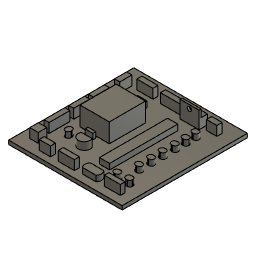
BIOGASMONITORING cad v0 (Autodesk Fusion 360 design; units mm, degrees)
Autodesk Fusion 360 part; units mm, degrees
sketch "Sketch1" plane through (0, 0, 0) normal (0, 1, 0) x (1, 0, 0)
  line L0 (25, 75) -> (85.032, 75)
  line L1 (85.032, 75) -> (85.032, 8.776)
  line L2 (85.032, 8.776) -> (25, 8.776)
  line L3 (25, 8.776) -> (25, 75)
  dimension "d1" = 60.032
  dimension "d2" = 66.224
  constraint horizontal L0
  constraint vertical L1
  constraint horizontal L2
  constraint vertical L3
  measures "d1" distance of L0.start L0.end
  measures "d2" distance of L0.start L2.end
extrude "Extrude1" add sketch "Sketch1" along normal blind 2
sketch "Sketch2" plane through (0, 2, 0) normal (0, 1, 0) x (-1, 0, 0)
  line L0 (-25, -8.776) -> (-85.032, -8.776)
  line L1 (-85.032, -8.776) -> (-85.032, -75)
  line L2 (-85.032, -75) -> (-25, -75)
  line L3 (-25, -75) -> (-25, -8.776)
  line L4 (-35.9338, -68.308) -> (-44.4138, -68.308)
  line L5 (-44.4138, -68.308) -> (-44.4138, -65.648)
  line L6 (-44.4138, -65.648) -> (-35.9338, -65.648)
  line L7 (-35.9338, -65.648) -> (-35.9338, -68.308)
  line L8 (-48.4167, -68.308) -> (-59.4367, -68.308)
  line L9 (-59.4367, -68.308) -> (-59.4367, -65.648)
  line L10 (-59.4367, -65.648) -> (-48.4167, -65.648)
  line L11 (-48.4167, -65.648) -> (-48.4167, -68.308)
  line L12 (-60.3881, -68.308) -> (-70.3881, -68.308)
  line L13 (-70.3881, -68.308) -> (-70.3881, -63.808)
  line L14 (-70.3881, -63.808) -> (-60.3881, -63.808)
  line L15 (-60.3881, -63.808) -> (-60.3881, -68.308)
  line L16 (-72.8571, -68.308) -> (-78.3401, -68.308)
  line L17 (-78.3401, -68.308) -> (-78.3401, -65.508)
  line L18 (-78.3401, -65.508) -> (-72.8571, -65.508)
  line L19 (-72.8571, -65.508) -> (-72.8571, -68.308)
  constraint horizontal L4
  constraint vertical L5
  constraint horizontal L6
  constraint vertical L7
  constraint horizontal L8
  constraint vertical L9
  constraint horizontal L10
  constraint vertical L11
  constraint horizontal L12
  constraint vertical L13
  constraint horizontal L14
  constraint vertical L15
  constraint horizontal L16
  constraint vertical L17
  constraint horizontal L18
  constraint vertical L19
extrude "Extrude2" add sketch "Sketch2" along normal blind 5 contours L4 L5 L6 L7 | L8 L9 L10 L11 | L16 L17 L18 L19
sketch "Sketch3" plane through (0, 2, 0) normal (0, 1, 0) x (-1, 0, 0)
  line L0 (-72.8571, -65.508) -> (-72.8571, -68.308)
  line L1 (-72.8571, -68.308) -> (-78.3401, -68.308)
  line L2 (-78.3401, -68.308) -> (-78.3401, -65.508)
  line L3 (-78.3401, -65.508) -> (-72.8571, -65.508)
  line L4 (-35.9338, -65.648) -> (-35.9338, -68.308)
  line L5 (-35.9338, -68.308) -> (-44.4138, -68.308)
  line L6 (-44.4138, -68.308) -> (-44.4138, -65.648)
  line L7 (-44.4138, -65.648) -> (-35.9338, -65.648)
  line L8 (-48.4167, -65.648) -> (-48.4167, -68.308)
  line L9 (-48.4167, -68.308) -> (-59.4367, -68.308)
  line L10 (-59.4367, -68.308) -> (-59.4367, -65.648)
  line L11 (-59.4367, -65.648) -> (-48.4167, -65.648)
  line L12 (-25, -8.776) -> (-85.032, -8.776)
  line L13 (-85.032, -8.776) -> (-85.032, -75)
  line L14 (-85.032, -75) -> (-25, -75)
  line L15 (-25, -75) -> (-25, -8.776)
  line L16 (-60.5977, -68.308) -> (-70.5977, -68.308)
  line L17 (-70.5977, -68.308) -> (-70.5977, -63.808)
  line L18 (-70.5977, -63.808) -> (-60.5977, -63.808)
  line L19 (-60.5977, -63.808) -> (-60.5977, -68.308)
  line L20 (-60.5977, -65.0802) -> (-70.5977, -65.0802)
  constraint horizontal L16
  constraint vertical L17
  constraint horizontal L18
  constraint vertical L19
  constraint coincident L19 L20.start
  constraint coincident L17 L20.end
  constraint perpendicular L17 L20
extrude "Extrude3" add sketch "Sketch3" along normal blind 5 contours L16 L17 L19 L20 | L17 L18 L19 L20
sketch "Sketch4" plane through (0, 7, 0) normal (0, 1, 0) x (-1, 0, 0)
  line L0 (-60.5977, -63.808) -> (-70.5977, -63.808)
  line L1 (-70.5977, -63.808) -> (-70.5977, -68.308)
  line L2 (-70.5977, -68.308) -> (-60.5977, -68.308)
  line L3 (-60.5977, -68.308) -> (-60.5977, -63.808)
  line L4 (-60.5977, -64.9469) -> (-70.5977, -64.9469)
  constraint coincident L3 L4.start
  constraint coincident L1 L4.end
  constraint perpendicular L1 L4
extrude "Extrude4" add sketch "Sketch4" along normal blind 4 contours L0 L1 L3 L4
sketch "Sketch5" plane through (0, 0, -64.9469) normal (0, 0, -1) x (-1, 0, 0)
  line L0 (-70.5977, 7) -> (-60.5977, 7)
  line L1 (-60.5977, 7) -> (-60.5977, 11)
  line L2 (-60.5977, 11) -> (-70.5977, 11)
  line L3 (-70.5977, 11) -> (-70.5977, 7)
  circle A0 centre (-65.5, 9) radius 1.118
extrude "Extrude5" cut sketch "Sketch5" against normal blind 1.5 contours A0
sketch "Sketch6" plane through (0, 2, 0) normal (0, 1, 0) x (-1, 0, 0)
  line L0 (-60.5977, -63.808) -> (-60.5977, -68.308)
  line L1 (-60.5977, -68.308) -> (-70.5977, -68.308)
  line L2 (-70.5977, -68.308) -> (-70.5977, -63.808)
  line L3 (-70.5977, -63.808) -> (-60.5977, -63.808)
  line L4 (-72.8571, -65.508) -> (-72.8571, -68.308)
  line L5 (-72.8571, -68.308) -> (-78.3401, -68.308)
  line L6 (-78.3401, -68.308) -> (-78.3401, -65.508)
  line L7 (-78.3401, -65.508) -> (-72.8571, -65.508)
  line L8 (-35.9338, -65.648) -> (-35.9338, -68.308)
  line L9 (-35.9338, -68.308) -> (-44.4138, -68.308)
  line L10 (-44.4138, -68.308) -> (-44.4138, -65.648)
  line L11 (-44.4138, -65.648) -> (-35.9338, -65.648)
  line L12 (-48.4167, -65.648) -> (-48.4167, -68.308)
  line L13 (-48.4167, -68.308) -> (-59.4367, -68.308)
  line L14 (-59.4367, -68.308) -> (-59.4367, -65.648)
  line L15 (-59.4367, -65.648) -> (-48.4167, -65.648)
  line L16 (-25, -8.776) -> (-85.032, -8.776)
  line L17 (-85.032, -8.776) -> (-85.032, -75)
  line L18 (-85.032, -75) -> (-25, -75)
  line L19 (-25, -75) -> (-25, -8.776)
  line L20 (-29.9588, -66.201) -> (-32.7588, -66.201)
  line L21 (-32.7588, -66.201) -> (-32.7588, -59.801)
  line L22 (-32.7588, -59.801) -> (-29.9588, -59.801)
  line L23 (-29.9588, -59.801) -> (-29.9588, -66.201)
  line L24 (-30, -54.417) -> (-32.66, -54.417)
  line L25 (-32.66, -54.417) -> (-32.66, -45.937)
  line L26 (-32.66, -45.937) -> (-30, -45.937)
  line L27 (-30, -45.937) -> (-30, -54.417)
  line L28 (-30, -44) -> (-32.66, -44)
  line L29 (-32.66, -44) -> (-32.66, -35.52)
  line L30 (-32.66, -35.52) -> (-30, -35.52)
  line L31 (-30, -35.52) -> (-30, -44)
  line L32 (-30, -33.528) -> (-32.66, -33.528)
  line L33 (-32.66, -33.528) -> (-32.66, -22.508)
  line L34 (-32.66, -22.508) -> (-30, -22.508)
  line L35 (-30, -22.508) -> (-30, -33.528)
  line L36 (-29.8577, -19.633) -> (-34.3577, -19.633)
  line L37 (-34.3577, -19.633) -> (-34.3577, -15.133)
  line L38 (-34.3577, -15.133) -> (-29.8577, -15.133)
  line L39 (-29.8577, -15.133) -> (-29.8577, -19.633)
  line L40 (-37.8047, -14.852) -> (-43.7447, -14.852)
  line L41 (-43.7447, -14.852) -> (-43.7447, -12.192)
  line L42 (-43.7447, -12.192) -> (-37.8047, -12.192)
  line L43 (-37.8047, -12.192) -> (-37.8047, -14.852)
  line L44 (-47.8727, -14.852) -> (-56.3527, -14.852)
  line L45 (-56.3527, -14.852) -> (-56.3527, -12.192)
  line L46 (-56.3527, -12.192) -> (-47.8727, -12.192)
  line L47 (-47.8727, -12.192) -> (-47.8727, -14.852)
  constraint horizontal L20
  constraint vertical L21
  constraint horizontal L22
  constraint vertical L23
  constraint horizontal L24
  constraint vertical L25
  constraint horizontal L26
  constraint vertical L27
  constraint horizontal L28
  constraint vertical L29
  constraint horizontal L30
  constraint vertical L31
  constraint horizontal L32
  constraint vertical L33
  constraint horizontal L34
  constraint vertical L35
  constraint horizontal L36
  constraint vertical L37
  constraint horizontal L38
  constraint vertical L39
  constraint horizontal L40
  constraint vertical L41
  constraint horizontal L42
  constraint vertical L43
  constraint horizontal L44
  constraint vertical L45
  constraint horizontal L46
  constraint vertical L47
extrude "Extrude6" add sketch "Sketch6" along normal blind 5 contours L20 L21 L22 L23 | L24 L25 L26 L27 | L28 L29 L30 L31 | L32 L33 L34 L35 | L36 L37 L38 L39 | L40 L41 L42 L43 | L44 L45 L46 L47
sketch "Sketch7" plane through (0, 2, 0) normal (0, 1, 0) x (-1, 0, 0)
  line L0 (-47.8727, -12.192) -> (-47.8727, -14.852)
  line L1 (-47.8727, -14.852) -> (-56.3527, -14.852)
  line L2 (-56.3527, -14.852) -> (-56.3527, -12.192)
  line L3 (-56.3527, -12.192) -> (-47.8727, -12.192)
  line L4 (-30, -35.52) -> (-30, -44)
  line L5 (-30, -44) -> (-32.66, -44)
  line L6 (-32.66, -44) -> (-32.66, -35.52)
  line L7 (-32.66, -35.52) -> (-30, -35.52)
  line L8 (-30, -45.937) -> (-30, -54.417)
  line L9 (-30, -54.417) -> (-32.66, -54.417)
  line L10 (-32.66, -54.417) -> (-32.66, -45.937)
  line L11 (-32.66, -45.937) -> (-30, -45.937)
  line L12 (-37.8047, -12.192) -> (-37.8047, -14.852)
  line L13 (-37.8047, -14.852) -> (-43.7447, -14.852)
  line L14 (-43.7447, -14.852) -> (-43.7447, -12.192)
  line L15 (-43.7447, -12.192) -> (-37.8047, -12.192)
  line L16 (-30, -22.508) -> (-30, -33.528)
  line L17 (-30, -33.528) -> (-32.66, -33.528)
  line L18 (-32.66, -33.528) -> (-32.66, -22.508)
  line L19 (-32.66, -22.508) -> (-30, -22.508)
  line L20 (-29.9588, -59.801) -> (-29.9588, -66.201)
  line L21 (-29.9588, -66.201) -> (-32.7588, -66.201)
  line L22 (-32.7588, -66.201) -> (-32.7588, -59.801)
  line L23 (-32.7588, -59.801) -> (-29.9588, -59.801)
  line L24 (-29.8577, -15.133) -> (-29.8577, -19.633)
  line L25 (-29.8577, -19.633) -> (-34.3577, -19.633)
  line L26 (-34.3577, -19.633) -> (-34.3577, -15.133)
  line L27 (-34.3577, -15.133) -> (-29.8577, -15.133)
  line L28 (-60.5977, -63.808) -> (-60.5977, -68.308)
  line L29 (-60.5977, -68.308) -> (-70.5977, -68.308)
  line L30 (-70.5977, -68.308) -> (-70.5977, -63.808)
  line L31 (-70.5977, -63.808) -> (-60.5977, -63.808)
  line L32 (-72.8571, -65.508) -> (-72.8571, -68.308)
  line L33 (-72.8571, -68.308) -> (-78.3401, -68.308)
  line L34 (-78.3401, -68.308) -> (-78.3401, -65.508)
  line L35 (-78.3401, -65.508) -> (-72.8571, -65.508)
  line L36 (-35.9338, -65.648) -> (-35.9338, -68.308)
  line L37 (-35.9338, -68.308) -> (-44.4138, -68.308)
  line L38 (-44.4138, -68.308) -> (-44.4138, -65.648)
  line L39 (-44.4138, -65.648) -> (-35.9338, -65.648)
  line L40 (-48.4167, -65.648) -> (-48.4167, -68.308)
  line L41 (-48.4167, -68.308) -> (-59.4367, -68.308)
  line L42 (-59.4367, -68.308) -> (-59.4367, -65.648)
  line L43 (-59.4367, -65.648) -> (-48.4167, -65.648)
  line L44 (-25, -8.776) -> (-85.032, -8.776)
  line L45 (-85.032, -8.776) -> (-85.032, -75)
  line L46 (-85.032, -75) -> (-25, -75)
  line L47 (-25, -75) -> (-25, -8.776)
  line L48 (-60.0787, -16.977) -> (-67.1737, -16.977)
  line L49 (-67.1737, -12.799) -> (-60.0787, -12.799)
  arc A0 (-60.0941, -16.977) -> (-60.0941, -12.799) centre (-61.8653, -14.888) ccw
  arc A1 (-67.1737, -12.799) -> (-67.1737, -16.977) centre (-64.9927, -14.888) ccw
  line L50 (-60.0787, -12.799) -> (-60.0787, -12.8122)
  line L51 (-60.0787, -16.9638) -> (-60.0787, -16.977)
  constraint horizontal L48
  constraint horizontal L49
  constraint vertical L50
  constraint coincident L48 A0.start
  constraint coincident L49 A0.end
  constraint coincident A0 L50.end
  constraint coincident A0 L51.start
  constraint collinear L50 L51
sketch "Sketch8" plane through (64.1506, 2, -14.888) normal (0, 1, 0) x (-1, 0, 0)
extrude "Extrude7" add sketch "Sketch7" along normal blind 3 contours L48 L49 A0 A1
sketch "Sketch9" plane through (0, 2, 0) normal (0, 1, 0) x (-1, 0, 0)
  line L0 (-60.0941, -16.977) -> (-67.1737, -16.977)
  arc A0 (-67.1737, -12.799) -> (-67.1737, -16.977) centre (-64.9927, -14.888) ccw
  line L1 (-67.1737, -12.799) -> (-60.0941, -12.799)
  arc A1 (-60.0941, -16.977) -> (-60.0941, -12.799) centre (-61.8653, -14.888) ccw
  line L2 (-47.8727, -12.192) -> (-47.8727, -14.852)
  line L3 (-47.8727, -14.852) -> (-56.3527, -14.852)
  line L4 (-56.3527, -14.852) -> (-56.3527, -12.192)
  line L5 (-56.3527, -12.192) -> (-47.8727, -12.192)
  line L6 (-30, -35.52) -> (-30, -44)
  line L7 (-30, -44) -> (-32.66, -44)
  line L8 (-32.66, -44) -> (-32.66, -35.52)
  line L9 (-32.66, -35.52) -> (-30, -35.52)
  line L10 (-30, -45.937) -> (-30, -54.417)
  line L11 (-30, -54.417) -> (-32.66, -54.417)
  line L12 (-32.66, -54.417) -> (-32.66, -45.937)
  line L13 (-32.66, -45.937) -> (-30, -45.937)
  line L14 (-37.8047, -12.192) -> (-37.8047, -14.852)
  line L15 (-37.8047, -14.852) -> (-43.7447, -14.852)
  line L16 (-43.7447, -14.852) -> (-43.7447, -12.192)
  line L17 (-43.7447, -12.192) -> (-37.8047, -12.192)
  line L18 (-30, -22.508) -> (-30, -33.528)
  line L19 (-30, -33.528) -> (-32.66, -33.528)
  line L20 (-32.66, -33.528) -> (-32.66, -22.508)
  line L21 (-32.66, -22.508) -> (-30, -22.508)
  line L22 (-29.9588, -59.801) -> (-29.9588, -66.201)
  line L23 (-29.9588, -66.201) -> (-32.7588, -66.201)
  line L24 (-32.7588, -66.201) -> (-32.7588, -59.801)
  line L25 (-32.7588, -59.801) -> (-29.9588, -59.801)
  line L26 (-29.8577, -15.133) -> (-29.8577, -19.633)
  line L27 (-29.8577, -19.633) -> (-34.3577, -19.633)
  line L28 (-34.3577, -19.633) -> (-34.3577, -15.133)
  line L29 (-34.3577, -15.133) -> (-29.8577, -15.133)
  line L30 (-60.5977, -63.808) -> (-60.5977, -68.308)
  line L31 (-60.5977, -68.308) -> (-70.5977, -68.308)
  line L32 (-70.5977, -68.308) -> (-70.5977, -63.808)
  line L33 (-70.5977, -63.808) -> (-60.5977, -63.808)
  line L34 (-72.8571, -65.508) -> (-72.8571, -68.308)
  line L35 (-72.8571, -68.308) -> (-78.3401, -68.308)
  line L36 (-78.3401, -68.308) -> (-78.3401, -65.508)
  line L37 (-78.3401, -65.508) -> (-72.8571, -65.508)
  line L38 (-35.9338, -65.648) -> (-35.9338, -68.308)
  line L39 (-35.9338, -68.308) -> (-44.4138, -68.308)
  line L40 (-44.4138, -68.308) -> (-44.4138, -65.648)
  line L41 (-44.4138, -65.648) -> (-35.9338, -65.648)
  line L42 (-48.4167, -65.648) -> (-48.4167, -68.308)
  line L43 (-48.4167, -68.308) -> (-59.4367, -68.308)
  line L44 (-59.4367, -68.308) -> (-59.4367, -65.648)
  line L45 (-59.4367, -65.648) -> (-48.4167, -65.648)
  line L46 (-25, -8.776) -> (-85.032, -8.776)
  line L47 (-85.032, -8.776) -> (-85.032, -75)
  line L48 (-85.032, -75) -> (-25, -75)
  line L49 (-25, -75) -> (-25, -8.776)
  line L50 (-71.3947, -12.799) -> (-79.8747, -12.799)
  line L51 (-79.8747, -12.799) -> (-79.8747, -15.459)
  line L52 (-79.8747, -15.459) -> (-71.3947, -15.459)
  line L53 (-71.3947, -15.459) -> (-71.3947, -12.799)
  line L54 (-75.325, -22.003) -> (-78.878, -22.003)
  line L55 (-78.878, -22.003) -> (-78.878, -18.955)
  line L56 (-78.878, -18.955) -> (-75.325, -18.955)
  line L57 (-75.325, -18.955) -> (-75.325, -22.003)
  constraint horizontal L50
  constraint vertical L51
  constraint horizontal L52
  constraint vertical L53
  constraint horizontal L54
  constraint vertical L55
  constraint horizontal L56
  constraint vertical L57
extrude "Extrude8" add sketch "Sketch9" along normal blind 3 contours L54 L55 L56 L57
fillet "Fillet1" radius 1.524 1 edges at (75.325, 3.5, -18.955)
fillet "Fillet2" radius 1.254 3 edges at (78.878, 3.5, -18.955) (78.878, 3.5, -22.003) (75.325, 3.5, -22.003)
sketch "Sketch10" plane through (0, 2, 0) normal (0, 1, 0) x (-1, 0, 0)
  line L0 (-75.325, -20.479) -> (-75.325, -20.749)
  arc A0 (-76.579, -22.003) -> (-75.325, -20.749) centre (-76.579, -20.749) ccw
  line L1 (-76.579, -22.003) -> (-77.624, -22.003)
  arc A1 (-78.878, -20.749) -> (-77.624, -22.003) centre (-77.624, -20.749) ccw
  line L2 (-78.878, -20.749) -> (-78.878, -20.209)
  arc A2 (-77.624, -18.955) -> (-78.878, -20.209) centre (-77.624, -20.209) ccw
  line L3 (-77.624, -18.955) -> (-76.849, -18.955)
  arc A3 (-75.325, -20.479) -> (-76.849, -18.955) centre (-76.849, -20.479) ccw
  line L4 (-60.0941, -16.977) -> (-67.1737, -16.977)
  arc A4 (-67.1737, -12.799) -> (-67.1737, -16.977) centre (-64.9927, -14.888) ccw
  line L5 (-67.1737, -12.799) -> (-60.0941, -12.799)
  arc A5 (-60.0941, -16.977) -> (-60.0941, -12.799) centre (-61.8653, -14.888) ccw
  line L6 (-47.8727, -12.192) -> (-47.8727, -14.852)
  line L7 (-47.8727, -14.852) -> (-56.3527, -14.852)
  line L8 (-56.3527, -14.852) -> (-56.3527, -12.192)
  line L9 (-56.3527, -12.192) -> (-47.8727, -12.192)
  line L10 (-30, -35.52) -> (-30, -44)
  line L11 (-30, -44) -> (-32.66, -44)
  line L12 (-32.66, -44) -> (-32.66, -35.52)
  line L13 (-32.66, -35.52) -> (-30, -35.52)
  line L14 (-30, -45.937) -> (-30, -54.417)
  line L15 (-30, -54.417) -> (-32.66, -54.417)
  line L16 (-32.66, -54.417) -> (-32.66, -45.937)
  line L17 (-32.66, -45.937) -> (-30, -45.937)
  line L18 (-37.8047, -12.192) -> (-37.8047, -14.852)
  line L19 (-37.8047, -14.852) -> (-43.7447, -14.852)
  line L20 (-43.7447, -14.852) -> (-43.7447, -12.192)
  line L21 (-43.7447, -12.192) -> (-37.8047, -12.192)
  line L22 (-30, -22.508) -> (-30, -33.528)
  line L23 (-30, -33.528) -> (-32.66, -33.528)
  line L24 (-32.66, -33.528) -> (-32.66, -22.508)
  line L25 (-32.66, -22.508) -> (-30, -22.508)
  line L26 (-29.9588, -59.801) -> (-29.9588, -66.201)
  line L27 (-29.9588, -66.201) -> (-32.7588, -66.201)
  line L28 (-32.7588, -66.201) -> (-32.7588, -59.801)
  line L29 (-32.7588, -59.801) -> (-29.9588, -59.801)
  line L30 (-29.8577, -15.133) -> (-29.8577, -19.633)
  line L31 (-29.8577, -19.633) -> (-34.3577, -19.633)
  line L32 (-34.3577, -19.633) -> (-34.3577, -15.133)
  line L33 (-34.3577, -15.133) -> (-29.8577, -15.133)
  line L34 (-60.5977, -63.808) -> (-60.5977, -68.308)
  line L35 (-60.5977, -68.308) -> (-70.5977, -68.308)
  line L36 (-70.5977, -68.308) -> (-70.5977, -63.808)
  line L37 (-70.5977, -63.808) -> (-60.5977, -63.808)
  line L38 (-72.8571, -65.508) -> (-72.8571, -68.308)
  line L39 (-72.8571, -68.308) -> (-78.3401, -68.308)
  line L40 (-78.3401, -68.308) -> (-78.3401, -65.508)
  line L41 (-78.3401, -65.508) -> (-72.8571, -65.508)
  line L42 (-35.9338, -65.648) -> (-35.9338, -68.308)
  line L43 (-35.9338, -68.308) -> (-44.4138, -68.308)
  line L44 (-44.4138, -68.308) -> (-44.4138, -65.648)
  line L45 (-44.4138, -65.648) -> (-35.9338, -65.648)
  line L46 (-48.4167, -65.648) -> (-48.4167, -68.308)
  line L47 (-48.4167, -68.308) -> (-59.4367, -68.308)
  line L48 (-59.4367, -68.308) -> (-59.4367, -65.648)
  line L49 (-59.4367, -65.648) -> (-48.4167, -65.648)
  line L50 (-25, -8.776) -> (-85.032, -8.776)
  line L51 (-85.032, -8.776) -> (-85.032, -75)
  line L52 (-85.032, -75) -> (-25, -75)
  line L53 (-25, -75) -> (-25, -8.776)
  line L54 (-71.3947, -15.459) -> (-79.8747, -15.459)
  line L55 (-79.8747, -15.459) -> (-79.8747, -13.003)
  line L56 (-79.8747, -13.003) -> (-71.3947, -13.003)
  line L57 (-71.3947, -13.003) -> (-71.3947, -15.459)
  line L58 (-72.969, -18.5676) -> (-69.416, -18.5676)
  line L59 (-72.969, -21.6156) -> (-72.969, -18.5676)
  line L60 (-69.416, -18.5676) -> (-69.416, -21.6156)
  line L61 (-69.416, -21.6156) -> (-72.969, -21.6156)
  line L62 (-71.623, -30.847) -> (-75.176, -30.847)
  line L63 (-75.176, -30.847) -> (-75.176, -27.799)
  line L64 (-75.176, -27.799) -> (-71.623, -27.799)
  line L65 (-71.623, -27.799) -> (-71.623, -30.847)
  line L66 (-71.623, -34.182) -> (-75.176, -34.182)
  line L67 (-75.176, -34.182) -> (-75.176, -37.23)
  line L68 (-75.176, -37.23) -> (-71.623, -37.23)
  line L69 (-71.623, -37.23) -> (-71.623, -34.182)
  line L70 (-75.176, -40.306) -> (-71.623, -40.306)
  line L71 (-71.623, -40.306) -> (-71.623, -43.354)
  line L72 (-71.623, -43.354) -> (-75.176, -43.354)
  line L73 (-75.176, -43.354) -> (-75.176, -40.306)
  line L74 (-71.623, -46.696) -> (-75.176, -46.696)
  line L75 (-75.176, -46.696) -> (-75.176, -49.744)
  line L76 (-71.623, -49.744) -> (-71.623, -46.696)
  line L77 (-71.623, -46.696) -> (-71.623, -49.744)
  line L78 (-71.623, -49.744) -> (-75.176, -49.744)
  line L79 (-75.176, -49.744) -> (-75.176, -46.696)
  line L80 (-71.623, -57.674) -> (-75.176, -57.674)
  line L81 (-75.176, -57.674) -> (-75.176, -60.722)
  line L82 (-75.176, -60.722) -> (-71.623, -60.722)
  line L83 (-71.623, -60.722) -> (-71.623, -57.674)
  line L84 (-71.623, -55.474) -> (-75.176, -55.474)
  line L85 (-75.176, -55.474) -> (-75.176, -52.426)
  line L86 (-75.176, -52.426) -> (-71.623, -52.426)
  line L87 (-71.623, -52.426) -> (-71.623, -55.474)
  constraint horizontal L54
  constraint vertical L55
  constraint horizontal L56
  constraint vertical L57
  constraint horizontal L61
  constraint vertical L59
  constraint horizontal L58
  constraint vertical L60
  constraint horizontal L62
  constraint vertical L63
  constraint horizontal L64
  constraint vertical L65
  constraint horizontal L66
  constraint vertical L67
  constraint horizontal L68
  constraint vertical L69
  constraint horizontal L70
  constraint vertical L71
  constraint horizontal L72
  constraint vertical L73
  constraint horizontal L74
  constraint vertical L75
  constraint vertical L76
  constraint vertical L77
  constraint horizontal L78
  constraint vertical L79
  constraint horizontal L80
  constraint vertical L81
  constraint horizontal L82
  constraint vertical L83
  constraint horizontal L84
  constraint vertical L85
  constraint horizontal L86
  constraint vertical L87
extrude "Extrude9" add sketch "Sketch10" along normal blind 3 contours L54 L55 L56 L57 | L58 L59 L60 L61 | L62 L63 L64 L65 | L66 L67 L68 L69 | L70 L71 L72 L73 | L74 L75 L76 L77 L78 L79 | L80 L81 L82 L83 | L84 L85 L86 L87
extrude "Extrude10" add 1 faces at (77.048, 5, -14.6403) along direction (0, 1, 0) blind 2
fillet "Fillet3" radius 1.524 4 edges at (69.416, 3.5, -18.5676) (69.416, 3.5, -21.6156) (72.969, 3.5, -18.5676) (72.969, 3.5, -21.6156)
fillet "Fillet4" radius 1.524 4 edges at (75.176, 3.5, -30.847) (71.623, 3.5, -30.847) (71.623, 3.5, -27.799) (75.176, 3.5, -27.799)
fillet "Fillet5" radius 1.524 4 edges at (71.623, 3.5, -34.182) (71.623, 3.5, -37.23) (75.176, 3.5, -37.23) (75.176, 3.5, -34.182)
fillet "Fillet6" radius 1.524 4 edges at (71.623, 3.5, -40.306) (71.623, 3.5, -43.354) (75.176, 3.5, -43.354) (75.176, 3.5, -40.306)
fillet "Fillet7" radius 1.524 4 edges at (75.176, 3.5, -46.696) (71.623, 3.5, -46.696) (75.176, 3.5, -49.744) (71.623, 3.5, -49.744)
fillet "Fillet8" radius 1.52 4 edges at (71.623, 3.5, -55.474) (71.623, 3.5, -52.426) (75.176, 3.5, -52.426) (75.176, 3.5, -55.474)
fillet "Fillet9" radius 1.524 4 edges at (75.176, 3.5, -57.674) (71.623, 3.5, -57.674) (75.176, 3.5, -60.722) (71.623, 3.5, -60.722)
sketch "Sketch11" plane through (0, 2, 0) normal (0, 1, 0) x (-1, 0, 0)
  line L0 (-71.3947, -13.003) -> (-71.3947, -15.459)
  line L1 (-71.3947, -15.459) -> (-79.8747, -15.459)
  line L2 (-79.8747, -15.459) -> (-79.8747, -13.003)
  line L3 (-79.8747, -13.003) -> (-71.3947, -13.003)
  line L4 (-73.652, -40.306) -> (-73.147, -40.306)
  arc A0 (-73.147, -43.354) -> (-73.147, -40.306) centre (-73.147, -41.83) ccw
  line L5 (-73.147, -43.354) -> (-73.652, -43.354)
  arc A1 (-73.652, -40.306) -> (-73.652, -43.354) centre (-73.652, -41.83) ccw
  line L6 (-73.147, -60.722) -> (-73.652, -60.722)
  arc A2 (-73.652, -57.674) -> (-73.652, -60.722) centre (-73.652, -59.198) ccw
  line L7 (-73.652, -57.674) -> (-73.147, -57.674)
  arc A3 (-73.147, -60.722) -> (-73.147, -57.674) centre (-73.147, -59.198) ccw
  line L8 (-73.147, -37.23) -> (-73.652, -37.23)
  arc A4 (-73.652, -34.182) -> (-73.652, -37.23) centre (-73.652, -35.706) ccw
  line L9 (-73.652, -34.182) -> (-73.147, -34.182)
  arc A5 (-73.147, -37.23) -> (-73.147, -34.182) centre (-73.147, -35.706) ccw
  line L10 (-70.94, -21.6156) -> (-71.445, -21.6156)
  arc A6 (-71.445, -18.5676) -> (-71.445, -21.6156) centre (-71.445, -20.0916) ccw
  line L11 (-71.445, -18.5676) -> (-70.94, -18.5676)
  arc A7 (-70.94, -21.6156) -> (-70.94, -18.5676) centre (-70.94, -20.0916) ccw
  line L12 (-73.147, -49.744) -> (-73.652, -49.744)
  arc A8 (-73.652, -46.696) -> (-73.652, -49.744) centre (-73.652, -48.22) ccw
  line L13 (-73.652, -46.696) -> (-73.147, -46.696)
  arc A9 (-73.147, -49.744) -> (-73.147, -46.696) centre (-73.147, -48.22) ccw
  line L14 (-71.623, -53.946) -> (-71.623, -53.954)
  arc A10 (-73.143, -55.474) -> (-71.623, -53.954) centre (-73.143, -53.954) ccw
  line L15 (-73.143, -55.474) -> (-73.656, -55.474)
  arc A11 (-75.176, -53.954) -> (-73.656, -55.474) centre (-73.656, -53.954) ccw
  line L16 (-75.176, -53.954) -> (-75.176, -53.946)
  arc A12 (-73.656, -52.426) -> (-75.176, -53.946) centre (-73.656, -53.946) ccw
  line L17 (-73.656, -52.426) -> (-73.143, -52.426)
  arc A13 (-71.623, -53.946) -> (-73.143, -52.426) centre (-73.143, -53.946) ccw
  arc A14 (-73.147, -30.847) -> (-73.147, -27.799) centre (-73.147, -29.323) ccw
  line L18 (-73.147, -30.847) -> (-73.652, -30.847)
  arc A15 (-73.652, -27.799) -> (-73.652, -30.847) centre (-73.652, -29.323) ccw
  line L19 (-73.652, -27.799) -> (-73.147, -27.799)
  line L20 (-75.325, -20.479) -> (-75.325, -20.749)
  arc A16 (-76.579, -22.003) -> (-75.325, -20.749) centre (-76.579, -20.749) ccw
  line L21 (-76.579, -22.003) -> (-77.624, -22.003)
  arc A17 (-78.878, -20.749) -> (-77.624, -22.003) centre (-77.624, -20.749) ccw
  line L22 (-78.878, -20.749) -> (-78.878, -20.209)
  arc A18 (-77.624, -18.955) -> (-78.878, -20.209) centre (-77.624, -20.209) ccw
  line L23 (-77.624, -18.955) -> (-76.849, -18.955)
  arc A19 (-75.325, -20.479) -> (-76.849, -18.955) centre (-76.849, -20.479) ccw
  line L24 (-60.0941, -16.977) -> (-67.1737, -16.977)
  arc A20 (-67.1737, -12.799) -> (-67.1737, -16.977) centre (-64.9927, -14.888) ccw
  line L25 (-67.1737, -12.799) -> (-60.0941, -12.799)
  arc A21 (-60.0941, -16.977) -> (-60.0941, -12.799) centre (-61.8653, -14.888) ccw
  line L26 (-47.8727, -12.192) -> (-47.8727, -14.852)
  line L27 (-47.8727, -14.852) -> (-56.3527, -14.852)
  line L28 (-56.3527, -14.852) -> (-56.3527, -12.192)
  line L29 (-56.3527, -12.192) -> (-47.8727, -12.192)
  line L30 (-30, -35.52) -> (-30, -44)
  line L31 (-30, -44) -> (-32.66, -44)
  line L32 (-32.66, -44) -> (-32.66, -35.52)
  line L33 (-32.66, -35.52) -> (-30, -35.52)
  line L34 (-30, -45.937) -> (-30, -54.417)
  line L35 (-30, -54.417) -> (-32.66, -54.417)
  line L36 (-32.66, -54.417) -> (-32.66, -45.937)
  line L37 (-32.66, -45.937) -> (-30, -45.937)
  line L38 (-37.8047, -12.192) -> (-37.8047, -14.852)
  line L39 (-37.8047, -14.852) -> (-43.7447, -14.852)
  line L40 (-43.7447, -14.852) -> (-43.7447, -12.192)
  line L41 (-43.7447, -12.192) -> (-37.8047, -12.192)
  line L42 (-30, -22.508) -> (-30, -33.528)
  line L43 (-30, -33.528) -> (-32.66, -33.528)
  line L44 (-32.66, -33.528) -> (-32.66, -22.508)
  line L45 (-32.66, -22.508) -> (-30, -22.508)
  line L46 (-29.9588, -59.801) -> (-29.9588, -66.201)
  line L47 (-29.9588, -66.201) -> (-32.7588, -66.201)
  line L48 (-32.7588, -66.201) -> (-32.7588, -59.801)
  line L49 (-32.7588, -59.801) -> (-29.9588, -59.801)
  line L50 (-29.8577, -15.133) -> (-29.8577, -19.633)
  line L51 (-29.8577, -19.633) -> (-34.3577, -19.633)
  line L52 (-34.3577, -19.633) -> (-34.3577, -15.133)
  line L53 (-34.3577, -15.133) -> (-29.8577, -15.133)
  line L54 (-60.5977, -63.808) -> (-60.5977, -68.308)
  line L55 (-60.5977, -68.308) -> (-70.5977, -68.308)
  line L56 (-70.5977, -68.308) -> (-70.5977, -63.808)
  line L57 (-70.5977, -63.808) -> (-60.5977, -63.808)
  line L58 (-72.8571, -65.508) -> (-72.8571, -68.308)
  line L59 (-72.8571, -68.308) -> (-78.3401, -68.308)
  line L60 (-78.3401, -68.308) -> (-78.3401, -65.508)
  line L61 (-78.3401, -65.508) -> (-72.8571, -65.508)
  line L62 (-35.9338, -65.648) -> (-35.9338, -68.308)
  line L63 (-35.9338, -68.308) -> (-44.4138, -68.308)
  line L64 (-44.4138, -68.308) -> (-44.4138, -65.648)
  line L65 (-44.4138, -65.648) -> (-35.9338, -65.648)
  line L66 (-48.4167, -65.648) -> (-48.4167, -68.308)
  line L67 (-48.4167, -68.308) -> (-59.4367, -68.308)
  line L68 (-59.4367, -68.308) -> (-59.4367, -65.648)
  line L69 (-59.4367, -65.648) -> (-48.4167, -65.648)
  line L70 (-25, -8.776) -> (-85.032, -8.776)
  line L71 (-85.032, -8.776) -> (-85.032, -75)
  line L72 (-85.032, -75) -> (-25, -75)
  line L73 (-25, -75) -> (-25, -8.776)
  line L74 (-60, -57.821) -> (-65.374, -57.821)
  line L75 (-65.374, -57.821) -> (-65.374, -21.821)
  line L76 (-65.374, -21.821) -> (-60, -21.821)
  line L77 (-60, -21.821) -> (-60, -57.821)
  line L78 (-41.578, -60.322) -> (-46.652, -60.322)
  line L79 (-46.652, -60.322) -> (-46.652, -58.798)
  line L80 (-46.652, -58.798) -> (-41.578, -58.798)
  line L81 (-41.578, -58.798) -> (-41.578, -60.322)
  line L82 (-41.589, -56.594) -> (-46.693, -56.594)
  line L83 (-46.693, -56.594) -> (-46.693, -54.294)
  line L84 (-46.693, -54.294) -> (-41.589, -54.294)
  line L85 (-41.589, -54.294) -> (-41.589, -56.594)
  line L86 (-37.798, -52.828) -> (-53.298, -52.828)
  line L87 (-53.298, -52.828) -> (-53.298, -33.728)
  line L88 (-53.298, -33.728) -> (-37.798, -33.728)
  line L89 (-37.798, -33.728) -> (-37.798, -52.828)
  line L90 (-37.35, -28.477) -> (-40.398, -28.477)
  line L91 (-40.398, -28.477) -> (-40.398, -24.924)
  line L92 (-40.398, -24.924) -> (-37.35, -24.924)
  line L93 (-37.35, -24.924) -> (-37.35, -28.477)
  line L94 (-43.089, -32.672) -> (-47.161, -32.672)
  line L95 (-47.161, -32.672) -> (-47.161, -31.148)
  line L96 (-47.161, -31.148) -> (-43.089, -31.148)
  line L97 (-43.089, -31.148) -> (-43.089, -32.672)
  line L98 (-44.5989, -27.556) -> (-50.4011, -27.556)
  arc A22 (-44.5989, -27.556) -> (-50.4011, -27.556) centre (-47.5, -26.2685) ccw
  dimension "d180" = 6.348
  constraint horizontal L74
  constraint vertical L75
  constraint horizontal L76
  constraint vertical L77
  constraint horizontal L78
  constraint vertical L79
  constraint horizontal L80
  constraint vertical L81
  constraint horizontal L82
  constraint vertical L83
  constraint horizontal L84
  constraint vertical L85
  constraint horizontal L86
  constraint vertical L87
  constraint horizontal L88
  constraint vertical L89
  constraint horizontal L90
  constraint vertical L91
  constraint horizontal L92
  constraint vertical L93
  constraint horizontal L94
  constraint vertical L95
  constraint horizontal L96
  constraint vertical L97
  constraint perpendicular L91 L98
  measures "d180" diameter of A22
extrude "Extrude11" add sketch "Sketch11" along normal blind 5 contours L74 L75 L76 L77 | L78 L79 L80 L81 | L82 L83 L84 L85 | L86 L87 L88 L89 | L90 L91 L92 L93 | L94 L95 L96 L97 | L98 A22
sketch "Sketch12" plane through (0, 7, 0) normal (0, 1, 0) x (-1, 0, 0)
  line L0 (-37.35, -24.924) -> (-40.398, -24.924)
  line L1 (-40.398, -24.924) -> (-40.398, -28.477)
  line L2 (-40.398, -28.477) -> (-37.35, -28.477)
  line L3 (-37.35, -28.477) -> (-37.35, -24.924)
extrude "Extrude12" cut sketch "Sketch12" against normal blind 2
fillet "Fillet10" radius 1.54 4 edges at (37.35, 3.5, -28.477) (37.35, 3.5, -24.924) (40.398, 3.5, -24.924) (40.398, 3.5, -28.477)
sketch "Sketch13" plane through (0, 7, 0) normal (0, 1, 0) x (-1, 0, 0)
  line L0 (-60, -21.821) -> (-65.374, -21.821)
  line L1 (-65.374, -21.821) -> (-65.374, -57.821)
  line L2 (-65.374, -57.821) -> (-60, -57.821)
  line L3 (-60, -57.821) -> (-60, -21.821)
extrude "Extrude13" cut sketch "Sketch13" against normal blind 2
sketch "Sketch14" plane through (0, 7, 0) normal (0, 1, 0) x (-1, 0, 0)
  line L0 (-37.798, -33.728) -> (-53.298, -33.728)
  line L1 (-53.298, -33.728) -> (-53.298, -52.828)
  line L2 (-53.298, -52.828) -> (-37.798, -52.828)
  line L3 (-37.798, -52.828) -> (-37.798, -33.728)
extrude "Extrude14" add sketch "Sketch14" along normal blind 5
sketch "Sketch15" plane through (0, 7, 0) normal (0, 1, 0) x (-1, 0, 0)
  line L0 (-43.089, -31.148) -> (-47.161, -31.148)
  line L1 (-47.161, -31.148) -> (-47.161, -32.672)
  line L2 (-47.161, -32.672) -> (-43.089, -32.672)
  line L3 (-43.089, -32.672) -> (-43.089, -31.148)
extrude "Extrude15" cut sketch "Sketch15" against normal blind 2
sketch "Sketch16" plane through (0, 7, 0) normal (0, 1, 0) x (-1, 0, 0)
  arc A0 (-44.5989, -27.556) -> (-50.4011, -27.556) centre (-47.5, -26.2685) ccw
  line L0 (-50.4011, -27.556) -> (-44.5989, -27.556)
extrude "Extrude16" cut sketch "Sketch16" against normal blind 1
sketch "Sketch17" plane through (0, 7, 0) normal (0, 1, 0) x (-1, 0, 0)
  line L0 (-41.589, -54.294) -> (-46.693, -54.294)
  line L1 (-46.693, -54.294) -> (-46.693, -56.594)
  line L2 (-46.693, -56.594) -> (-41.589, -56.594)
  line L3 (-41.589, -56.594) -> (-41.589, -54.294)
extrude "Extrude17" cut sketch "Sketch17" 1 faces at (44.9607, 7, -59.814) against normal blind 2
